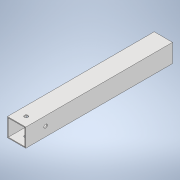
# Autodesk Inventor part: 4_barra
Saved by Autodesk Inventor 2020 (Build 240168000, 168)
## iProperties
Created: 2019-10-11
Part Number: 4_barra
Material: Generico
Document SubType Name: Modeling
Designer: socci
Density: 1 g/cm^3
Appearance: Default
Author: socci
Autodesk Inventor part; units mm, degrees
ref_plane "YZ Plane" through (0, 0, 0) normal (1, 0, 0) x (0, 1, 0)
ref_plane "XZ Plane" through (0, 0, 0) normal (0, 1, 0) x (-1, 0, 0)
ref_plane "XY Plane" through (0, 0, 0) normal (0, 0, 1) x (1, 0, 0)
sketch "Schizzo1" plane through (0, 0, 0) normal (0, 0, 1) x (1, 0, 0)
  line L0 (12.5, -12.5) -> (-12.5, -12.5)
  line L1 (-12.5, -12.5) -> (-12.5, 12.5)
  line L2 (-12.5, 12.5) -> (12.5, 12.5)
  line L3 (12.5, 12.5) -> (12.5, -12.5)
  line L4 (11.3, 11.3) -> (-11.3, 11.3)
  line L5 (-11.3, 11.3) -> (-11.3, -11.3)
  line L6 (-11.3, -11.3) -> (11.3, -11.3)
  line L7 (11.3, -11.3) -> (11.3, 11.3)
  point P0 (0, 0)
  point P1 (0, 0)
  dimension "d0" = 25
  dimension "d1" = 1.2
  constraints: 16 end point, 1 coincident, 12 other
  measures "d0" distance of L1.end L2.end
  measures "d1" distance between parallel lines of L2 L4
extrude "Estrusione1" add sketch "Schizzo1" against normal blind 200
sketch "Schizzo2" plane through (-12.5, 12.5, 0) normal (0, 1, 0) x (1, 0, 0)
  circle A0 centre (12.5, 13) radius 2.5 projected
  point P0 (12.5, 0)
hole "Foro1" at (0, 12.5, -13) direction (0, -1, 0) diameter 5 end through all
sketch "Schizzo3" plane through (12.5, -12.5, 0) normal (1, 0, 0) x (0, 0, -1)
  circle A0 centre (27, 12.5) radius 2.5 projected
  point P0 (0, 12.5)
hole "Foro2" at (12.5, 0, -27) direction (-1, 0, 0) diameter 5 end through all
